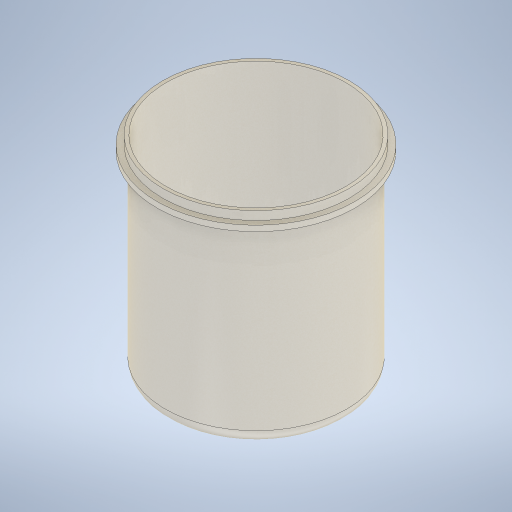
# Autodesk Inventor part: ContenedorTest
Saved by Autodesk Inventor 2024 (Build 280153000, 153)
## iProperties
Created: 2024-05-15
Part Number: ContenedorTest
Material: Genérico
Document SubType Name: Modeling
Designer: alexa
Density: 1 g/cm^3
Appearance: Valor por defecto
Author: alexa
Autodesk Inventor part; units mm, degrees
ref_plane "YZ Plane" through (0, 0, 0) normal (1, 0, 0) x (0, 1, 0)
ref_plane "XZ Plane" through (0, 0, 0) normal (0, 1, 0) x (-1, 0, 0)
ref_plane "XY Plane" through (0, 0, 0) normal (0, 0, 1) x (1, 0, 0)
sketch "Sketch1" plane through (0, 0, 0) normal (0, 0, 1) x (1, 0, 0)
  line L0 (46.8, 0) -> (47.9667, 0)
  line L1 (47.9667, 7.5) -> (47.9667, 101.6997)
  line L2 (47.725, 109.1997) -> (47.525, 109.1997)
  line L3 (47.525, 109.1997) -> (47.525, 7.7)
  line L4 (47.525, 109.1997) -> (49.325, 109.1997)
  line L5 (49.325, 109.1997) -> (49.325, 104.6997)
  line L6 (49.325, 104.6997) -> (52.325, 104.6997)
  line L7 (52.325, 104.6997) -> (52.325, 101.6997)
  line L8 (52.325, 101.6997) -> (49.325, 101.6997)
  line L9 (49.325, 101.6997) -> (47.9667, 101.6997)
  line L10 (0, 0) -> (0, 20.8136)
  line L11 (40.4667, 0) -> (-0.2292, 0)
  line L12 (0, 0) -> (0, 0.2)
  line L13 (0, 0.2) -> (40.025, 0.2)
  arc A0 (40.025, 0.2) -> (47.525, 7.7) centre (40.025, 7.7) ccw
  arc A1 (40.4667, 0) -> (47.9667, 7.5) centre (40.4667, 7.5) ccw
  dimension "d1" = 0.2
  dimension "d2" = 109.2
  dimension "d3" = 1.8
  dimension "d4" = 4.5
  dimension "d5" = 3
  dimension "d6" = 3
  dimension "d7" = 0.2
  dimension "d8" = 90
  dimension "d14" = 7.5
  dimension "d15" = 0.2
  constraints: 28 end point, 5 perpendicular, 5 point on line, 4 point on circle, 4 tangent, 3 horizontal, 2 centre point, 2 parallel, 1 equal radius, 1 vertical
  measures "d1" distance of L2.end L2.start
  measures "d2" distance of L2.start L0.end
  measures "d3" distance of L2.end L4.end
  measures "d4" distance of L4.end L5.end
  measures "d5" distance of L5.end L6.end
  measures "d6" distance of L6.end L7.end
  measures "d7" distance of L10.start L12.end
  measures "d8" angle of L12 L13
  measures "d14" radius of A1
  measures "d15" vertical distance of A1.centre A0.centre
revolve "Revolution1" add sketch "Sketch1" angle 360 about axis through (0, 0, 0) along (0, 1, 0)
sketch "Sketch2" plane through (0, 0, 0) normal (0, -1, 0) x (1, 0, 0)
  circle A0 centre (0, 0) radius 6.8
  dimension "d11" = 13.6
  constraints: 1 centre point, 1 coincident
  measures "d11" diameter of A0
extrude "Extrusion1" cut sketch "Sketch2" against normal blind 1
sketch "Sketch3" plane through (0, 0, 0) normal (0, -1, 0) x (1, 0, 0)
  circle A0 centre (0, 0) radius 37.85
  circle A1 centre (0, 0) radius 6.8 projected
  circle A2 centre (0, 0) radius 39.5
  dimension "d16" = 75.7
  dimension "d17" = 79
  constraints: 2 centre point, 2 coincident
  measures "d16" diameter of A0
  measures "d17" diameter of A2
extrude "Extrusion2" add sketch "Sketch3" along normal blind 2 contours A2
body "Solid1"
